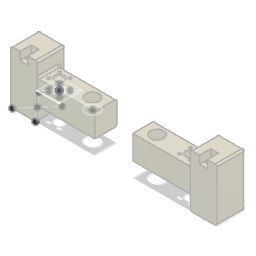
FinalCSProject2 v8 (Autodesk Fusion 360 design; units mm, degrees)
Autodesk Fusion 360 part; units mm, degrees
note: some values were not read from the file. Set by a fixed rule: which sketch regions a step uses.
sketch "Sketch1" plane through (0, 0, 0) normal (0, 1, 0) x (1, 0, 0)
  circle A0 centre (0, 0) radius 5.5
  line L0 (-12.5, 12.5) -> (12.5, 12.5)
  line L1 (12.5, 12.5) -> (12.5, -12.5)
  line L2 (12.5, -12.5) -> (-12.5, -12.5)
  line L3 (-12.5, -12.5) -> (-12.5, 12.5)
  line L4 (-12.5, 12.5) -> (12.5, -12.5) construction
  line L5 (12.5, 12.5) -> (-12.5, -12.5) construction
  line L6 (-12.5, -12.5) -> (12.5, 12.5) construction
  line L7 (0, 0) -> (0, 6) construction
  line L8 (0, 6) -> (6, 6) construction
  line L9 (0, 6) -> (-6, 6) construction
  line L10 (6, 6) -> (6, -6) construction
  line L11 (6, -6) -> (-6, -6) construction
  line L12 (-6, 6) -> (-6, -6) construction
  circle A1 centre (-6, 6) radius 1.6
  circle A2 centre (6, 6) radius 1.6
  circle A3 centre (6, -6) radius 1.6
  circle A4 centre (-6, -6) radius 1.6
  line L13 (0, 0) -> (37.5, 0)
  circle A5 centre (37.5, 0) radius 7.5
  dimension "d1" = 11
  dimension "d2" = 25
  dimension "d3" = 25
  dimension "d4" = 6
  dimension "d5" = 6
  dimension "d6" = 6
  dimension "d7" = 12
  dimension "d8" = 12
  dimension "d14" = 3.2
  dimension "d15" = 3.2
  dimension "d16" = 3.2
  dimension "d17" = 3.2
  dimension "d92" = 37.5
  dimension "d93" = 15
  constraint coincident A0.centre L7.start
  constraint horizontal L0
  constraint perpendicular L0 L1
  constraint parallel L0 L2
  constraint parallel L1 L3
  constraint coincident L4 A0.centre
  constraint coincident L5 A0.centre
  constraint vertical L7
  constraint perpendicular L7 L8
  constraint perpendicular L7 L9
  constraint coincident L4 L10.end
  constraint perpendicular L10 L11
  constraint coincident L9.end L12.start
  constraint coincident L8.end L10.start
  constraint coincident L10.end L11.start
  constraint coincident L11.end L12.end
  constraint perpendicular L7 L13
  constraint coincident L13.end A5.centre
  measures "d1" diameter of A0
  measures "d2" distance of L1.end L2.end
  measures "d3" distance of L0.end L1.end
  measures "d4" distance of A0.centre L7.end
  measures "d5" distance of L7.end L8.end
  measures "d6" distance of L7.end L9.end
  measures "d7" distance of L8.end L10.end
  measures "d8" distance of L10.end L11.end
  measures "d14" diameter of A1
  measures "d15" diameter of A2
  measures "d16" diameter of A3
  measures "d17" diameter of A4
  measures "d92" distance of A0.centre L13.end
  measures "d93" diameter of A5
extrude "Extrude1" add sketch "Sketch1" along normal blind 2 contours L0 L1 L2 L3 makes body 1
extrude "Extrude2" add 1 faces at (-1.8052, 0, -10.8298) along direction (0, -1, 0) blind 10 on bodies 1 bodies 1
sketch "Sketch3" plane through (0, -10, 0) normal (0, -1, 0) x (1, 0, 0)
  circle A0 centre (0, 0) radius 5.5
  circle A1 centre (-6, -6) radius 1.6
  circle A2 centre (6, 6) radius 1.6
  circle A3 centre (-6, 6) radius 1.6
  circle A4 centre (6, -6) radius 1.6
  line L0 (12.5, 12.5) -> (-12.5, 12.5)
  line L1 (-12.5, 12.5) -> (-12.5, -12.5)
  line L2 (-12.5, -12.5) -> (12.5, -12.5)
  line L3 (12.5, -12.5) -> (12.5, 12.5)
  line L4 (-12.5, 12.5) -> (12.5, -12.5) construction
  line L5 (12.5, 12.5) -> (-12.5, -12.5) construction
  circle A5 centre (0, 0) radius 4.5
  circle A6 centre (6, 6) radius 2.5
  circle A7 centre (6, -6) radius 2.5
  circle A8 centre (-6, -6) radius 2.5
  circle A9 centre (-6, 6) radius 2.5
  dimension "d22" = 9
  dimension "d23" = 5
  dimension "d24" = 5
  dimension "d25" = 5
  dimension "d26" = 5
  constraint coincident L0.end L1.start
  constraint coincident L2.end L3.start
  constraint coincident L0.start L3.end
  constraint coincident L1.end L2.start
  constraint coincident A0.centre A5.centre
  constraint concentric A2 A6
  constraint concentric A4 A7
  constraint concentric A1 A8
  constraint concentric A3 A9
  measures "d22" diameter of A5
  measures "d23" diameter of A6
  measures "d24" diameter of A7
  measures "d25" diameter of A8
  measures "d26" diameter of A9
extrude "Extrude3" add 1 faces at (-1.8052, 2, -10.8298) along direction (0, 1, 0) blind 10 on bodies 1 bodies 1
extrude "Extrude4" add sketch "Sketch3" along normal blind 5 contours A0 | L0 L1 L2 L3 bodies 1
sketch "Sketch4" plane through (-12.5, 0, 0) normal (-1, 0, 0) x (0, 0, 1)
  line L0 (-12.5, 12) -> (-12.5, -15)
  line L1 (-12.5, -15) -> (12.5, -15)
  line L2 (12.5, -15) -> (12.5, 12)
  line L3 (12.5, 12) -> (-12.5, 12)
  line L4 (12.3812, 23.5) -> (-12.3812, 23.5)
  line L5 (-12.3812, 23.5) -> (-12.3812, -26.5)
  line L6 (-12.3812, -26.5) -> (12.3812, -26.5)
  line L7 (12.3812, -26.5) -> (12.3812, 23.5)
  line L8 (12.3812, 23.5) -> (-12.3812, -26.5) construction
  line L9 (-12.3812, 23.5) -> (12.3812, -26.5) construction
  point P0 (0, -1.5)
  dimension "d39" = 50
  constraint horizontal L4
  constraint perpendicular L4 L5
  constraint parallel L4 L6
  constraint parallel L5 L7
  constraint coincident L8 P0
  constraint coincident L9 P0
  measures "d39" distance of L4.end L5.end
extrude "Extrude5" add sketch "Sketch4" along normal blind 25 contours L3 L4 L5 L7 | L1 L3 L5 L7 | L1 L5 L6 L7 bodies 1
sketch "Sketch5" plane through (0, 0, -12.3812) normal (0, 0, -1) x (-1, 0, 0)
  line L0 (12.5, 23.5) -> (12.5, 12)
  line L1 (12.5, 12) -> (12.5, -15)
  line L2 (12.5, -26.5) -> (37.5, -26.5)
  line L3 (37.5, -26.5) -> (37.5, 23.5)
  line L4 (37.5, 23.5) -> (12.5, 23.5)
  line L5 (12.5, -15) -> (12.5, -26.5)
extrude "Extrude6" add sketch "Sketch5" along normal blind 2.038 bodies 1
extrude "Extrude7" add 1 faces at (-37.5, -9.8333, 3.4477) along direction (-1, 0, 0) blind 5 on bodies 1 bodies 1
extrude "Extrude8" add 1 faces at (-22.5, -26.5, -5.4857) along direction (0, -1, 0) blind 5 on bodies 1 bodies 1
extrude "Extrude9" add 1 faces at (-22.5, 23.5, -5.4857) along direction (0, 1, 0) blind 5 on bodies 1 bodies 1
extrude "Extrude10" add 1 faces at (-32.5, 8.5, -14.4192) along direction (0, 0, -1) blind 5.081 on bodies 1 bodies 1
sketch "Sketch7" plane through (0, 0, -19.5002) normal (0, 0, -1) x (-1, 0, 0)
  line L0 (12.5, 28.5) -> (12.5, -31.5)
  line L1 (12.5, -31.5) -> (42.5, -31.5)
  line L2 (42.5, -31.5) -> (42.5, 28.5)
  line L3 (42.5, 28.5) -> (12.5, 28.5)
  line L4 (12.5, 28.5) -> (42.5, -31.5) construction
  line L5 (12.5, -31.5) -> (42.5, 28.5) construction
  line L6 (38.5, 19.5) -> (16.5, 19.5)
  line L7 (16.5, 19.5) -> (16.5, -22.5)
  line L8 (16.5, -22.5) -> (38.5, -22.5)
  line L9 (38.5, -22.5) -> (38.5, 19.5)
  line L10 (38.5, 19.5) -> (16.5, -22.5) construction
  line L11 (16.5, 19.5) -> (38.5, -22.5) construction
  line L12 (38.5, 25.5) -> (16.5, 25.5) construction
  line L13 (16.5, 25.5) -> (16.5, -28.5) construction
  line L14 (16.5, -28.5) -> (38.5, -28.5) construction
  line L15 (38.5, -28.5) -> (38.5, 25.5) construction
  line L16 (38.5, 25.5) -> (16.5, -28.5) construction
  line L17 (16.5, 25.5) -> (38.5, -28.5) construction
  line L18 (16.5, 19.5) -> (16.5, 22.5) construction
  line L19 (38.5, 19.5) -> (38.5, 22.5) construction
  line L20 (16.5, 22.5) -> (38.5, 22.5) construction
  line L21 (27.5, 25.5) -> (27.5, 19.5) construction
  line L22 (27.5, 19.5) -> (22.5, 19.5) construction
  line L23 (22.5, 19.5) -> (22.5, 22.5) construction
  line L24 (27.5, 19.5) -> (32.5, 19.5) construction
  line L25 (32.5, 19.5) -> (32.5, 22.5) construction
  circle A0 centre (22.5, 22.5) radius 2
  circle A1 centre (32.5, 22.5) radius 2
  line L26 (27.5, -22.5) -> (27.5, -28.5) construction
  line L27 (27.5, -22.5) -> (32.5, -22.5) construction
  line L28 (27.5, -22.5) -> (22.5, -22.5) construction
  line L29 (32.5, -22.5) -> (32.5, -25.5) construction
  line L30 (22.5, -22.5) -> (22.5, -25.5) construction
  circle A2 centre (22.5, -25.5) radius 2
  circle A3 centre (32.5, -25.5) radius 2 construction
  circle A4 centre (32.5, -25.5) radius 2
  point P0 (27.5, -1.5)
  point P1 (27.5, -1.5)
  dimension "d54" = 22
  dimension "d55" = 42
  dimension "d56" = 22
  dimension "d57" = 54
  dimension "d58" = 3
  dimension "d59" = 3
  dimension "d60" = 5
  dimension "d61" = 5
  dimension "d62" = 4
  dimension "d63" = 4
  dimension "d64" = 5
  dimension "d65" = 5
  dimension "d66" = 3
  dimension "d67" = 3
  dimension "d68" = 4
  dimension "d69" = 4
  constraint coincident L0.start L3.end
  constraint coincident L1.end L2.start
  constraint coincident L0.end L1.start
  constraint coincident L2.end L3.start
  constraint horizontal L6
  constraint perpendicular L6 L7
  constraint parallel L6 L8
  constraint parallel L7 L9
  constraint coincident L10 P1
  constraint coincident L11 P1
  constraint midpoint L4 P1
  constraint horizontal L12
  constraint perpendicular L12 L13
  constraint parallel L12 L14
  constraint parallel L13 L15
  constraint coincident L16 P1
  constraint coincident L17 P1
  constraint coincident P1 P0
  constraint perpendicular L6 L18
  constraint perpendicular L6 L19
  constraint midpoint L12 L21.start
  constraint midpoint L6 L21.end
  constraint perpendicular L21 L22
  constraint coincident L20 L23.end
  constraint perpendicular L20 L23
  constraint perpendicular L21 L24
  constraint coincident L20 L25.end
  constraint perpendicular L20 L25
  constraint coincident L23.end A0.centre
  constraint coincident L25.end A1.centre
  constraint midpoint L8 L26.start
  constraint midpoint L14 L26.end
  constraint perpendicular L26 L27
  constraint perpendicular L26 L28
  constraint perpendicular L27 L29
  constraint perpendicular L28 L30
  constraint coincident L30.end A2.centre
  constraint coincident L29.end A3.centre
  constraint concentric A3 A4
  measures "d54" distance of L7.end L8.end
  measures "d55" distance of L6.end L7.end
  measures "d56" distance of L13.end L14.end
  measures "d57" distance of L12.end L13.end
  measures "d58" distance of L6.end L18.end
  measures "d59" distance of L6.start L19.end
  measures "d60" distance of L21.end L22.end
  measures "d61" distance of L21.end L24.end
  measures "d62" diameter of A0
  measures "d63" diameter of A1
  measures "d64" distance of L26.start L27.end
  measures "d65" distance of L26.start L28.end
  measures "d66" distance of L27.end L29.end
  measures "d67" distance of L28.end L30.end
  measures "d68" diameter of A2
  measures "d69" diameter of A3
extrude "Extrude11" cut sketch "Sketch7" against normal blind 27 contours L6 L7 L8 L9 bodies 1
extrude "Extrude12" cut sketch "Sketch7" against normal blind 10 contours A0 bodies 1
extrude "Extrude13" cut sketch "Sketch7" against normal blind 10 contours A1 bodies 1
extrude "Extrude14" cut sketch "Sketch7" against normal blind 10 contours A4 bodies 1
extrude "Extrude15" cut sketch "Sketch7" against normal blind 10 contours A2 bodies 1
extrude "Extrude18" add 1 faces at (-32.5, 3, 12.3812) along direction (0, 0, 1) blind 0.119 on bodies 1 bodies 1
fillet "Fillet5" radius 2 13 edges at (-27.5, -31.5, -19.5002) (-42.5, -1.5, -19.5002) (-12.5, -1.5, -19.5002) (-27.5, 28.5, -19.5002) (-12.5, -31.5, -3.5) (-42.5, -31.5, -3.5) (0, -15, -12.5) (-12.5, -1.5, -12.5) (-12.5, -15, 0) (0, 12, -12.5) (-12.5, 12, 0) (-12.5, 28.5, -3.5) (-42.5, 28.5, -3.5) on bodies 1
sketch "Sketch8" plane through (0, 28.5, 0) normal (0, 1, 0) x (-1, 0, 0)
  line L0 (40.5, -17.5002) -> (40.5, 12.5002)
  line L1 (40.5, 12.5002) -> (14.5, 12.5002)
  line L2 (14.5, 12.5002) -> (14.5, -17.5002)
  line L3 (14.5, -17.5002) -> (40.5, -17.5002)
  line L4 (12.5, 12.5, -2) -> (42.5, -19.5, -2)
  line L5 (12.5, -19.5, -2) -> (42.5, 12.5, -2)
  line L6 (27.5, -3.5, -2) -> (27.5, 12.5002, 0) construction
  line L7 (23, 0) -> (32, 0)
  line L8 (32, 0) -> (32, 25.0004)
  line L9 (32, 25.0004) -> (23, 25.0004)
  line L10 (23, 25.0004) -> (23, 0)
  line L11 (23, 0) -> (32, 25.0004) construction
  line L12 (32, 0) -> (23, 25.0004) construction
  point P0 (27.5, 12.5002)
  constraint midpoint L1 P0
  constraint horizontal L7
  constraint perpendicular L7 L8
  constraint parallel L7 L9
  constraint parallel L8 L10
  constraint coincident L11 P0
  constraint coincident L12 P0
extrude "Extrude19" cut sketch "Sketch8" against normal blind 9 contours L1 L7 L8 L10 bodies 1
extrude "Extrude20" add 1 faces at (12.5, -5.3333, 4.1667) along direction (1, 0, 0) blind 25 on bodies 1 bodies 1
extrude "Extrude21" add 1 faces at (37.5, -5.3333, 4.1667) along direction (1, 0, 0) blind 15 on bodies 1 bodies 1
extrude "Extrude22" cut sketch "Sketch1" along normal blind 100 and the other way blind 100 contours A5 bodies 1
sketch "Sketch9" plane through (0, -31.5, 0) normal (0, -1, 0) x (1, 0, 0)
  line L0 (-40.5, 12.5002) -> (-40.5, -17.5002)
  line L1 (-40.5, -17.5002) -> (-14.5, -17.5002)
  line L2 (-14.5, -17.5002) -> (-14.5, 12.5002)
  line L3 (-14.5, 12.5002) -> (-40.5, 12.5002)
  line L4 (-40.5, 12.5002) -> (-14.5, -17.5002)
  line L5 (-14.5, 12.5002) -> (-40.5, -17.5002)
  point P0 (-27.5, -2.5)
  constraint coincident L0.start L3.end
  constraint coincident L1.end L2.start
  constraint coincident L2.end L3.start
  constraint coincident L0.end L1.start
  constraint midpoint L5 P0
ref_plane "WorkPlane1" through (74, 0, 0) normal (1, 0, 0) x (0, 1, 0)
mirror "Mirror1" about plane through (74, 0, 0) normal (1, 0, 0) of bodies 1 makes body 2
